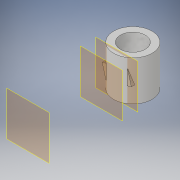
# Autodesk Inventor part: Propeller
Saved by Autodesk Inventor 2017 (Build 210142000, 142)
## iProperties
Created: 2018-05-10
Part Number: Propeller
Material: Generic
Document SubType Name: Modeling
Designer: Kyle
Density: 1 g/cm^3
Appearance: Default
Author: Kyle
Autodesk Inventor part; units mm, degrees
ref_plane "YZ Plane" through (0, 0, 0) normal (1, 0, 0) x (0, 1, 0)
ref_plane "XZ Plane" through (0, 0, 0) normal (0, 1, 0) x (-1, 0, 0)
sketch "Sketch1" plane through (0, 0, 0) normal (0, 1, 0) x (-1, 0, 0)
  circle A0 centre (0, 0) radius 2.4498
  circle A1 centre (0, 0) radius 3.791
  dimension "d0" = 4.8997
  dimension "d8" = 7.5819
  constraints: 2 centre point, 2 coincident
  measures "d0" diameter of A0
  measures "d8" diameter of A1
extrude "Extrusion1" add sketch "Sketch1" along normal blind 7.9045
ref_plane "Work Plane1" through (0, 0, 3.175) normal (0, 0, 1) x (1, 0, 0)
sketch "Sketch2" plane through (0, 0, 3.175) normal (0, 0, 1) x (1, 0, 0)
  line L0 (3.791, 7.9045) -> (-3.791, 7.9045) construction
  line L1 (0, 7.9045) -> (0, 0) construction
  line L2 (-2.8757, 4.6253) -> (-2.1539, 1.9315)
  line L3 (-2.1539, 1.9315) -> (2.8757, 3.2791)
  line L4 (2.8757, 3.2791) -> (2.1539, 5.973)
  line L5 (2.1539, 5.973) -> (-2.8757, 4.6253)
  line L6 (-2.8757, 4.6253) -> (2.8757, 3.2791) construction
  line L7 (-2.1539, 1.9315) -> (2.1539, 5.973) construction
  line L8 (-2.8757, 4.6253) -> (-0.0868, 4.6253) construction
  point P0 (0, 3.9522)
  dimension "d12" = 2.7889
  dimension "d13" = 75
  dimension "d14" = 5.207
  constraints: 16 end point, 4 midpoint, 2 parallel, 1 equal length, 1 horizontal, 1 perpendicular, 1 vertical
  measures "d12" distance of L2.start L2.end
  measures "d13" angle of L2 L8
  measures "d14" distance of L3.end L2.end
ref_plane "Work Plane3" through (0, 0, 20.7391) normal (0, 0, 1) x (1, 0, 0)
ref_plane "Work Plane2" through (0, 0, 6.2255) normal (0, 0, 1) x (1, 0, 0)
extrude "Extrusion2" add sketch "Sketch2" against normal blind 0.635
equation "\"d1\" = 7.7978"
equation "\"d2\" = 3.23596"
equation "\"d3\" = 9.60882"
equation "\"d4\" = 4.89966"
equation "\"d5\" = 1.98374"
equation "\"d6\" = 1.4732"
equation "\"d7\" = 1.23952"
body "Solid1"
